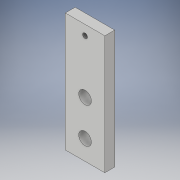
# Autodesk Inventor part: ShoulderScrewHolderSlide
Saved by Autodesk Inventor 2017 (Build 210142000, 142)
## iProperties
Created: 2017-12-26
Part Number: ShoulderScrewHolderSlide
Material: Generic
Document SubType Name: Modeling
Designer: User
Density: 1 g/cm^3
Appearance: Default
Author: User
Autodesk Inventor part; units mm, degrees
ref_plane "YZ Plane" through (0, 0, 0) normal (1, 0, 0) x (0, 1, 0)
ref_plane "XZ Plane" through (0, 0, 0) normal (0, 1, 0) x (-1, 0, 0)
ref_plane "XY Plane" through (0, 0, 0) normal (0, 0, 1) x (1, 0, 0)
sketch "Sketch1" plane through (0, 0, 0) normal (0, 0, 1) x (1, 0, 0)
  line L0 (0, 0) -> (12.7, 0)
  line L1 (12.7, 0) -> (12.7, 38.1)
  line L2 (12.7, 38.1) -> (0, 38.1)
  line L3 (0, 38.1) -> (0, 0)
  dimension "d0" = 12.7
  dimension "d1" = 38.1
  constraints: 8 end point, 2 parallel, 1 horizontal, 1 perpendicular
  measures "d0" distance of L2.end L1.end
  measures "d1" distance of L1.end L0.end
extrude "Extrusion1" add sketch "Sketch1" along normal blind 3.175
sketch "Sketch2" plane through (0, 0, 3.175) normal (0, 0, 1) x (1, 0, 0)
  line L0 (0, 34.925) -> (6.35, 34.925)
  line L1 (12.7, 38.1) -> (0, 38.1) projected
  point P0 (6.35, 4.445)
  dimension "d23" = 3.175
  constraints: 2 end point, 1 coincident, 1 horizontal
  measures "d23" distance from line of L1 point (6.35, 34.925)
hole "Hole1" at (6.35, 34.925, 3.175) direction (0, 0, -1) diameter 1.5748 end through all
sketch "Sketch3" plane through (0, 0, 3.175) normal (0, 0, 1) x (1, 0, 0)
  line L0 (12.7, 0) -> (12.7, 38.1) projected
  line L1 (0, 0) -> (12.7, 0) projected
  line L2 (0, 38.1) -> (0, 0) projected
  line L3 (0, 6.35) -> (6.35, 6.35)
  line L4 (6.35, 6.35) -> (6.35, 17.78)
  dimension "d24" = 6.35
  dimension "d25" = 6.35
  dimension "d26" = 11.43
  constraints: 4 end point, 2 coincident, 1 perpendicular, 1 point on line, 1 vertical
  measures "d24" distance of L3.start L3.end
  measures "d25" distance between parallel lines of L1 L3
  measures "d26" distance of L4.start L4.end
hole "Hole3" at (6.35, 6.35, 3.175) at (6.35, 17.78, 3.175) direction (0, 0, -1) diameter 4.064 depth 25.4 tip angle 118
body "Solid1"
